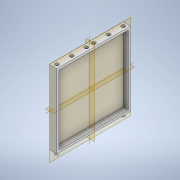
# Autodesk Inventor part: Wall
Saved by Autodesk Inventor 2022.4 (Build 264492010, 492A)
## iProperties
Created: 2025-02-20
Part Number: Wall
Material: Generic
Document SubType Name: Modeling
Designer: jan-m
Density: 1 g/cm^3
Appearance: Default
Author: jan-m
Autodesk Inventor part; units mm, degrees
sketch "Sketch2" plane through (0, 0, 0) normal (1, 0, 0) x (0, 1, 0)
  line L0 (50, 50) -> (-50, 50)
  line L1 (-50, 50) -> (-50, -50)
  line L2 (-50, -50) -> (50, -50)
  line L3 (50, -50) -> (50, 50)
  line L4 (-70, 0) -> (70, 0) projected
  line L5 (0, 70) -> (0, -70) projected
  point P0 (0, 0)
  point P1 (50, 0)
  point P2 (0, 50)
  dimension "d0" = 100
  dimension "d1" = 100
  constraints: 8 end point, 2 midpoint, 2 parallel, 2 point on line, 1 horizontal, 1 perpendicular
  measures "d0" distance of L2.end L0.start
  measures "d1" distance of L1.end L2.end
extrude "Extrusion1" add sketch "Sketch2" along normal mid plane 10
sketch "Sketch3" plane through (5, 0, 0) normal (1, 0, 0) x (0, 0, -1)
  line L0 (-47, 47) -> (47, 47)
  line L1 (47, 47) -> (47, -47)
  line L2 (47, -47) -> (-47, -47)
  line L3 (-47, -47) -> (-47, 47)
  line L4 (0, -70) -> (0, 70) projected
  line L5 (-70, 0) -> (70, 0) projected
  point P0 (0, 0)
  point P1 (0, 47)
  point P2 (-47, 0)
  dimension "d4" = 94
  dimension "d5" = 94
  constraints: 8 end point, 2 midpoint, 2 parallel, 2 point on line, 1 horizontal, 1 perpendicular
  measures "d4" distance of L0.start L0.end
  measures "d5" distance of L0.end L1.end
extrude "Extrusion2" cut sketch "Sketch3" against normal blind 7
sketch "Sketch5" plane through (-5, 50, 50) normal (0, 1, 0) x (1, 0, 0)
  circle A0 centre (5, 5) radius 2.5
  line L0 (10, 0) -> (0, 0) projected
  line L1 (5, 120) -> (5, -20) projected
  circle A1 centre (5, 25) radius 2.5
  circle A2 centre (5, 45) radius 2.5
  circle A3 centre (5, 95) radius 2.5
  line L2 (0, 100) -> (10, 100) projected
  circle A4 centre (5, 75) radius 2.5
  circle A5 centre (5, 55) radius 2.5
  point P0 (5, 50)
  dimension "d26" = 5
  dimension "d27" = 5
  dimension "d30" = 20
  dimension "d35" = 5
  dimension "d36" = 5
  dimension "d39" = 20
  constraints: 6 centre point, 2 point on line, 2 vertical, 8 other
  measures "d26" diameter of A0
  measures "d27" distance from line of L0 A0.centre
  measures "d30" distance of A0.centre A1.centre
  measures "d35" diameter of A3
  measures "d36" distance from line of L2 A3.centre
  measures "d39" distance of A3.centre A4.centre
extrude "Extrusion3" cut sketch "Sketch5" against normal blind 7
sketch "Sketch6" plane through (-5, -50, -50) normal (0, -1, 0) x (1, 0, 0)
  circle A0 centre (5, 95) radius 2.5
  line L0 (0, 100) -> (10, 100) projected
  line L1 (5, -20) -> (5, 120) projected
  line L2 (5, 120) -> (5, -20) projected
  line L3 (0, 0) -> (10, 0) projected
  line L4 (-2, 50) -> (12, 50) projected
  circle A1 centre (5, 5) radius 2.5
  point P0 (5, 50)
  dimension "d46" = 5
  dimension "d47" = 5
  constraints: 2 centre point, 1 point on line, 1 symmetric about line, 1 other
  measures "d46" diameter of A0
  measures "d47" distance from line of L0 A0.centre
extrude "Extrusion4" add sketch "Sketch6" along normal blind 5
body "Solid1"
